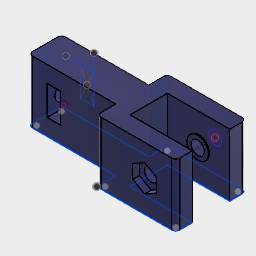
x-axis_tensioning_arm_for_toothed_idlers (Autodesk Fusion 360 design; units mm, degrees)
Autodesk Fusion 360 part; units mm, degrees
sketch "Skizze1" plane through (0, 0, 0) normal (0, 1, 0) x (1, 0, 0)
  line L0 (0.9885, -0.5) -> (20.9885, -0.5)
  line L1 (25, 0) -> (25, -9)
  line L2 (20.9885, -8.5) -> (0.9885, -8.5)
  line L3 (-0.0115, -7.5) -> (-0.0115, -1.5)
  arc A0 (0.9885, -0.5) -> (-0.0115, -1.5) centre (0.9885, -1.5) ccw
  line L4 (25, 0) -> (40, 0)
  line L5 (40, 0) -> (40, 3)
  line L6 (39, 4) -> (21.9885, 4)
  line L7 (20.9885, 3) -> (20.9885, -0.5)
  line L8 (25, -9) -> (40, -9)
  line L9 (40, -9) -> (40, -12)
  line L10 (39, -13) -> (21.9885, -13)
  line L11 (20.9885, -12) -> (20.9885, -8.5)
  arc A1 (20.9885, -12) -> (21.9885, -13) centre (21.9885, -12) ccw
  arc A2 (40, 3) -> (39, 4) centre (39, 3) ccw
  arc A3 (21.9885, 4) -> (20.9885, 3) centre (21.9885, 3) ccw
  arc A4 (39, -13) -> (40, -12) centre (39, -12) ccw
  arc A5 (-0.0115, -7.5) -> (0.9885, -8.5) centre (0.9885, -7.5) ccw
  dimension "d1" = 1
  dimension "d5" = 1
  dimension "d6" = 1
  dimension "d7" = 1
  dimension "d8" = 1
  dimension "d9" = 1
  dimension "d17" = 15
  dimension "d33" = 9
  dimension "d34" = 6
  dimension "d35" = 3
  dimension "d44" = 20
  constraint horizontal L0
  constraint vertical L1
  constraint horizontal L2
  constraint vertical L3
  constraint tangent L0 A0
  constraint tangent L3 A0
  constraint horizontal L4
  constraint vertical L5
  constraint horizontal L6
  constraint vertical L7
  constraint horizontal L8
  constraint vertical L9
  constraint horizontal L10
  constraint vertical L11
  constraint coincident origin L10
  constraint coincident origin L11
  constraint tangent L10 A1
  constraint tangent L11 A1
  constraint tangent L5 A2
  constraint tangent L6 A2
  constraint tangent L6 A3
  constraint tangent L7 A3
  constraint tangent L9 A4
  constraint tangent L10 A4
  constraint tangent L2 A5
  constraint tangent L3 A5
  constraint equal L4 L8
  constraint equal L7 L11
  constraint equal L5 L9
  constraint equal L0 L2
  measures "d1" radius of A0
  measures "d5" radius of A1
  measures "d6" radius of A2
  measures "d7" radius of A3
  measures "d8" radius of A4
  measures "d9" radius of A5
  measures "d33" distance of origin
  measures "d34" distance of origin
  measures "d35" distance of origin
extrude "Extrusion1" add sketch "Skizze1" along normal blind 15
sketch "Skizze6" plane through (0, 0, 13) normal (0, 0, 1) x (1, 0, 0)
  line L0 (21.9885, 0) -> (39, 0)
  line L1 (39, 0) -> (39, 15)
  line L2 (39, 15) -> (21.9885, 15)
  line L3 (21.9885, 15) -> (21.9885, 0)
  line L4 (25, 15) -> (40, 15)
  line L5 (25, 0) -> (40, 0)
  circle A0 centre (32.5, 7.5) radius 1.6
  line L6 (35.3537, 9.1391) -> (32.5074, 10.7909)
  line L7 (32.5074, 10.7909) -> (29.6537, 9.1518)
  line L8 (29.6537, 9.1518) -> (29.6463, 5.8609)
  line L9 (29.6463, 5.8609) -> (32.4927, 4.2091)
  line L10 (32.4927, 4.2091) -> (35.3463, 5.8482)
  line L11 (35.3463, 5.8482) -> (35.3537, 9.1391)
  dimension "d18" = 3.2
  dimension "d60" = 5.7
  measures "d18" diameter of A0
  measures "d60" distance of L8 L11
extrude "Extrusion4" cut sketch "Skizze6" against normal blind 1.6 contours L6 L7 L8 L9 L10 L11
extrude "Extrusion5" cut sketch "Skizze6" against normal blind 4 contours A0
sketch "Skizze9" plane through (0, 0, -4) normal (0, 0, -1) x (-1, 0, 0)
  line L0 (-39, 0) -> (-21.9885, 0)
  line L1 (-21.9885, 0) -> (-21.9885, 15)
  line L2 (-21.9885, 15) -> (-39, 15)
  line L3 (-39, 15) -> (-39, 0)
  circle A0 centre (-32.5, 7.5) radius 1.6
  circle A1 centre (-32.5, 7.5) radius 1.6
  measures "d5" radius of origin
hole "Bohrung2" at (32.5, 7.5, -4) direction (0, 0, 1) diameter 3.2 depth 4 tip angle 180 counterbore diameter 6 counterbore depth 1
cylinder "Grundkörper Zylinder1" add diameter 5.2 height 0.2 placed x (0, 1, 0) y (1, 0, 0) z (0, 0, -1) at (32.5, 7.5, 9)
extrude "Extrusion6" cut sketch "Skizze6" against normal blind 4.2 contours A0
cylinder "Grundkörper Zylinder2" add diameter 5.2 height 0.2 placed x (1, 0, 0) y (0, 1, 0) z (0, 0, 1) at (32.5, 7.5, 0)
extrude "Extrusion7" cut sketch "Skizze9" against normal blind 4.2 contours A0 A1
sketch "Skizze12" plane through (-0.0115, 0, 0) normal (-1, 0, 0) x (0, 0, 1)
  line L0 (1.5, 0) -> (7.5, 0)
  line L1 (7.5, 0) -> (7.5, 15)
  line L2 (7.5, 15) -> (1.5, 15)
  line L3 (1.5, 15) -> (1.5, 0)
  circle A0 centre (4.5, 7.5) radius 2.1
  dimension "d45" = 4.2
  measures "d45" diameter of A0
extrude "Extrusion8" cut sketch "Skizze12" against normal blind 18 contours A0
sketch "Skizze13" plane through (0, 0, 0.5) normal (0, 0, -1) x (-1, 0, 0)
  line L0 (-20.9885, 0) -> (-0.9885, 0)
  line L1 (-0.9885, 0) -> (-0.9885, 15)
  line L2 (-0.9885, 15) -> (-20.9885, 15)
  line L3 (-20.9885, 15) -> (-20.9885, 0)
  line L4 (-4.4885, 3.95) -> (-7.7885, 3.95)
  line L5 (-7.7885, 3.95) -> (-7.7885, 11.05)
  line L6 (-7.7885, 11.05) -> (-4.4885, 11.05)
  line L7 (-4.4885, 11.05) -> (-4.4885, 3.95)
  line L8 (-4.4885, 3.95) -> (-7.7885, 11.05) construction
  line L9 (-7.7885, 3.95) -> (-4.4885, 11.05) construction
  line L10 (-4.4885, 11.05) -> (-0.9885, 11.05)
  line L11 (-7.7885, 11.05) -> (-7.7885, 15)
  dimension "d52" = 7.1
  dimension "d53" = 3.3
  dimension "d54" = 3.5
  dimension "d55" = 3.95
  constraint perpendicular L4 L5
  constraint parallel L4 L6
  constraint parallel L5 L7
  constraint horizontal L4
  constraint coincident L8 origin
  constraint coincident L9 origin
  constraint coincident L1 origin
  constraint perpendicular L1 L10
  constraint vertical L11
  constraint coincident L2 origin
  measures "d52" distance of origin
extrude "Extrusion10" cut sketch "Skizze6" against normal blind 1.5 contours L6 L7 L8 L9 L10 L11
extrude "Extrusion9" cut sketch "Skizze13" against normal blind 8 contours L4 L5 L6 L7
